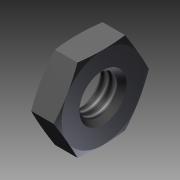
# Autodesk Inventor part: 205-S-M
Saved by Autodesk Inventor 2011 SP1 (Build 150282100, 282)
## iProperties
Created: 2017-03-01
Part Number: 205-S-M
Catalog Web Link: www.cadenas.de
Description: MU-SU-Mutter
Vendor: DESTACO
Document SubType Name: Modeling
Designer: psAdmin
Manufacturer: DESTACO
Mass: 0.073274 g
Surface Area: 1.37832 cm^2
Volume: 0.073274 cm^3
Density: 1 g/cm^3
Category: PARTsolutions
Company: DESTACO
Title: 205-S-M
Author: Cadenas PARTsolutions
Comments: Mutter
PSOL_IDENT_0: {$CADENAS_DATA\23d-libs\destaco\destaco_gmbh\man_spann\horizontalspanner\standard\su_parts\mutter_su
PSOL_IDENT_1: .prj},157 {VTYP=3D},{NB=205-S-M},{LINA=205-S-M},{NN=MU-SU},{DATE=20.09.2016 07:53:12},{GEOMDATE=08.1
PSOL_IDENT_2: 2.2009 09:59:00},{VERSION=v1},{LINEID=20},{LINESUBID=-1},{WBVAR=}  {NB=205-S-M},{LINA=205-S-M},{KT=D
PSOL_IDENT_3: UMMY},{MODELL=205-S-M},{SIZE=1},{MOD=1.000}
NN: MU-SU
NT: Mutter
NB: 205-S-M
NBSYN: $MODELL.
LINA: 205-S-M
MODELL: 205-S-M
SIZE: 1
MOD: 1.000
SUPPLIER: DESTACO
ARTICLENO: 205-S-M
BOMINFO: 205-S-M
CREATOR: CADENAS GmbH
Autodesk Inventor part; units mm, degrees
sketch "Skizze_1" plane through (0, 0, 0) normal (0, 1, 0) x (-1, 0, 0)
  line L0 (-3.749, 0) -> (-1.549, 0)
  line L1 (-1.549, 0) -> (-1.549, -3.5)
  line L2 (-1.549, -3.5) -> (-2.649, -7.6053)
  line L3 (-2.649, -7.6053) -> (-3.749, -3.5)
  line L4 (-3.749, -3.5) -> (-3.749, 0)
  line L5 (-3.749, 0) -> (-1.549, 0)
  constraints: 12 end point
revolve "Revolution1" add sketch "Skizze_1" angle 360 about axis through (3.749, 0, 0) along (1, 0, 0)
sketch "Skizze_2" plane through (0, 0, 0) normal (1, 0, 0) x (0, 1, 0)
  line L0 (-35, 26) -> (-35, -52)
  line L1 (-35, -52) -> (26, -52)
  line L2 (26, -52) -> (26, 26)
  line L3 (26, 26) -> (-35, 26)
  line L4 (-2.0207, 3.5) -> (-4.0415, 0)
  line L5 (-4.0415, 0) -> (-2.0207, -3.5)
  line L6 (-2.0207, -3.5) -> (2.0207, -3.5)
  line L7 (2.0207, -3.5) -> (4.0415, 0)
  line L8 (4.0415, 0) -> (2.0207, 3.5)
  line L9 (2.0207, 3.5) -> (-2.0207, 3.5)
  constraints: 20 end point
extrude "Extrusion1" cut sketch "Skizze_2" along normal blind 10
sketch "Skizze_3" plane through (0, 0, 0) normal (0, 1, 0) x (-1, 0, 0)
  line L0 (-3.749, 0) -> (-1.549, 0)
  line L1 (-1.549, 0) -> (-1.549, -2)
  line L2 (-1.549, -2) -> (-1.928, -1.621)
  line L3 (-1.928, -1.621) -> (-3.37, -1.621)
  line L4 (-3.37, -1.621) -> (-3.749, -2)
  line L5 (-3.749, -2) -> (-3.749, 0)
  line L6 (-3.749, 0) -> (-1.549, 0)
  constraints: 14 end point
revolve "Revolution2" cut sketch "Skizze_3" angle 360 about axis through (3.749, 0, 0) along (1, 0, 0)
thread "Thread1" size "M4x0.7" class "6H" standard "ISO Metric profile" full length
ref_plane "M_XY" through (0, 0, 0) normal (1, 0, 0) x (0, 0, -1)
ref_plane "M_YZ" through (0, 0, 0) normal (0, 0, -1) x (0, 1, 0)
ref_plane "M_ZX" through (0, 0, 0) normal (0, 1, 0) x (1, 0, 0)
body "Solid1"
